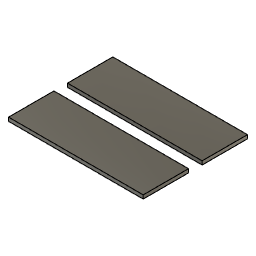
_BaseKhangFLora.5a7b964b-473b-4ecd-a55c-78e90f2e57d4 (Autodesk Fusion 360 design; units mm, degrees)
Autodesk Fusion 360 part; units mm, degrees
sketch "Sketch3" plane through (0, 0, 0) normal (0, 0, 1) x (1, 0, 0)
  line L0 (74.25, 25) -> (-74.25, 25)
  line L1 (-74.25, 25) -> (-74.25, -25)
  line L2 (-74.25, -25) -> (74.25, -25)
  line L3 (74.25, -25) -> (74.25, 25)
  line L4 (74.25, 25) -> (-74.25, -25) construction
  line L5 (-74.25, 25) -> (74.25, -25) construction
  dimension "d8" = 50
  dimension "d9" = 148.5
  constraint perpendicular L0 L1
  constraint parallel L0 L2
  constraint parallel L1 L3
  constraint horizontal L0
  constraint coincident L4 origin
  constraint coincident L5 origin
  measures "d8" distance of L0.end L1.end
  measures "d9" distance of L0.start L0.end
extrude "Extrude4" add sketch "Sketch3" along normal blind 4 makes body 1
copy_body "CopyPasteBodies1" bodies 1 makes body 2
move_body "Move1" bodies 2 to x (1, 0, 0) y (0, 1, 0) z (0, 0, 1) at (0, 65, 0)
